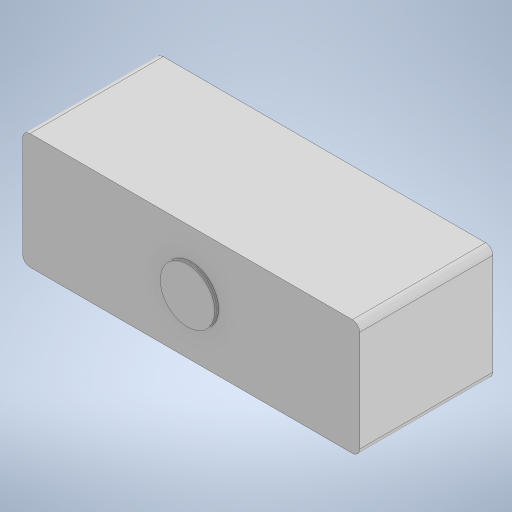
# Autodesk Inventor part: zed_x_mini
Saved by Autodesk Inventor 2024.3 (Build 283343010, 343A)
## iProperties
Created: 2025-07-19
Part Number: zed_x_mini
Material: 一般
Document SubType Name: Modeling
Designer: hikou
Density: 1 g/cm^3
Appearance: 既定
Author: hikou
Autodesk Inventor part; units mm, degrees
ref_plane "YZ Plane" through (0, 0, 0) normal (1, 0, 0) x (0, 1, 0)
ref_plane "XZ Plane" through (0, 0, 0) normal (0, 1, 0) x (-1, 0, 0)
ref_plane "XY Plane" through (0, 0, 0) normal (0, 0, 1) x (1, 0, 0)
sketch "スケッチ2" plane through (0, 0, 0) normal (0, 0, 1) x (1, 0, 0)
  line L0 (-46.15, -15.85) -> (46.15, -15.85)
  line L1 (46.15, -15.85) -> (46.15, 15.85)
  line L2 (46.15, 15.85) -> (-46.15, 15.85)
  line L3 (-46.15, 15.85) -> (-46.15, -15.85)
  line L4 (-46.15, -15.85) -> (46.15, 15.85) construction
  line L5 (46.15, -15.85) -> (-46.15, 15.85) construction
  point P0 (0, 0)
  dimension "d4" = 92.3
  dimension "d5" = 31.7
  constraints: 12 end point, 2 midpoint, 2 parallel, 1 horizontal, 1 perpendicular
  measures "d4" distance of L2.end L1.end
  measures "d5" distance of L1.end L0.end
extrude "押し出し2" add sketch "スケッチ2" along normal mid plane 36.5
fillet "フィレット1" radius 2 4 edges at (46.15, 15.85, 0) (46.15, -15.85, 0) (-46.15, 15.85, 0) (-46.15, -15.85, 0)
sketch "スケッチ3" plane through (-44.15, -15.85, -18.25) normal (0, -1, 0) x (1, 0, 0)
  line L0 (-2, 36.5) -> (-2, 0) projected
  line L1 (0, 36.5) -> (88.3, 36.5) projected
  point P0 (44.15, 18.25)
  point P1 (44.15, 21)
  dimension "d9" = 46.15
  dimension "d10" = 15.5
  measures "d9" distance from line of L0 point (44.15, 21)
  measures "d10" distance from line of L1 point (44.15, 21)
hole "穴1" at (0, -15.85, 2.75) direction (0, 1, 0) diameter 4.9784 depth 19.05 tip angle 118 thread size "1/4-20 UNC" class "2B" standard "ANSI Unified Screw Threads"
sketch "スケッチ4" plane through (0, 0, 18.25) normal (0, 0, 1) x (1, 0, 0)
  circle A0 centre (0, 0) radius 7.5
  dimension "d18" = 15
  constraints: 1 centre point, 1 coincident
  measures "d18" diameter of A0
extrude "押し出し3" add sketch "スケッチ4" along normal blind 1
